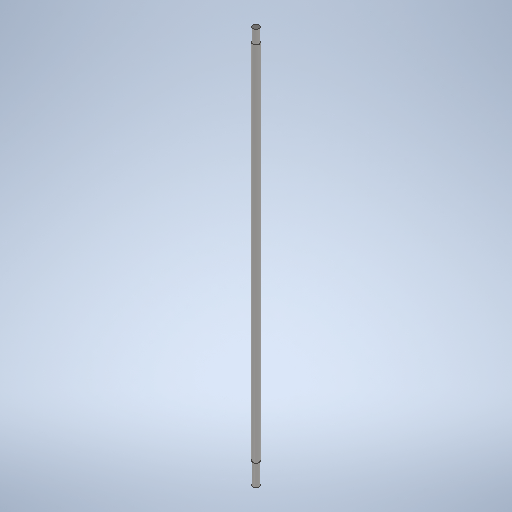
# Autodesk Inventor part: Eixotrifilado
Saved by Autodesk Inventor 2025 (Build 290162010, 162A)
## iProperties
Created: 2024-10-15
Part Number: Eixotrifilado
Material: Steel, Alloy
Document SubType Name: Modeling
Designer: Bryan Ss
Mass: 442.637 g
Surface Area: 230.763 cm^2
Volume: 57.2622 cm^3
Density: 7.73 g/cm^3
Appearance: Semi-Polished
Author: Bryan Ss
Autodesk Inventor part; units mm, degrees
ref_plane "YZ Plane" through (0, 0, 0) normal (1, 0, 0) x (0, 1, 0)
ref_plane "XZ Plane" through (0, 0, 0) normal (0, 1, 0) x (-1, 0, 0)
ref_plane "XY Plane" through (0, 0, 0) normal (0, 0, 1) x (1, 0, 0)
sketch "Sketch4" plane through (0, 0, 0) normal (0, 1, 0) x (-1, 0, 0)
  circle A0 centre (0, 0) radius 6.35
  dimension "d10" = 12.7
  constraints: 1 centre point, 1 coincident
  measures "d10" diameter of A0
extrude "Extrusion4" add sketch "Sketch4" along normal blind 745
sketch "Sketch5" plane through (0, 745, 0) normal (0, 1, 0) x (1, 0, 0)
  circle A0 centre (0, 0) radius 5.95
  circle A1 centre (0, 0) radius 6.35
  dimension "d13" = 11.9
  constraints: 2 centre point, 2 coincident
  measures "d13" diameter of A0
extrude "Extrusion5" cut sketch "Sketch5" against normal blind 25
sketch "Sketch6" plane through (0, 0, 0) normal (0, -1, 0) x (1, 0, 0)
  circle A0 centre (0, 0) radius 6.35 projected
  circle A1 centre (0, 0) radius 5.95 projected
extrude "Extrusion6" cut sketch "Sketch6" against normal blind 40
body "Solid2"
